Autodesk Fusion 360 part; units mm, degrees
(part 6 of 13)
  line L4448 (118.391, -108.231) -> (118.395, -108.209)
  line L4449 (123.628, -105.486) -> (123.648, -105.363)
  line L4450 (118.413, -108.169) -> (118.428, -108.142)
  line L4451 (133.306, -110.097) -> (133.194, -110.04)
  line L4452 (134.009, -109.5) -> (133.915, -109.438)
  line L4453 (133.194, -110.04) -> (133.106, -109.952)
  line L4454 (124.028, -105.086) -> (124.152, -105.106)
  line L4455 (133.665, -110.04) -> (133.553, -110.097)
  line L4456 (133.753, -109.952) -> (133.665, -110.04)
  line L4457 (119.458, -107.165) -> (123.205, -107.165)
  line L4458 (133.049, -109.84) -> (133.029, -109.717)
  line L4459 (133.194, -109.393) -> (133.306, -109.336)
  line L4460 (123.648, -105.363) -> (123.705, -105.251)
  line L4461 (134.224, -109.549) -> (134.224, -109.544)
  line L4462 (133.765, -109.235) -> (133.742, -109.183)
  line L4463 (134.144, -109.542) -> (134.009, -109.5)
  line L4464 (133.915, -109.438) -> (133.79, -109.553)
  line L4465 (133.106, -109.952) -> (133.049, -109.84)
  line L4466 (134.724, -109.549) -> (134.224, -109.549)
  line L4467 (133.029, -109.717) -> (133.049, -109.593)
  line L4468 (123.793, -105.163) -> (123.905, -105.106)
  line L4469 (133.049, -109.593) -> (133.106, -109.481)
  line L4470 (133.62, -109.37) -> (133.765, -109.235)
  line L4471 (133.553, -110.097) -> (133.429, -110.117)
  line L4472 (133.429, -110.117) -> (133.306, -110.097)
  line L4473 (133.829, -109.717) -> (133.81, -109.84)
  line L4474 (118.571, -110.489) -> (118.459, -110.433)
  line L4475 (133.81, -109.84) -> (133.753, -109.952)
  line L4476 (134.224, -109.544) -> (134.144, -109.542)
  line L4477 (133.106, -109.481) -> (133.194, -109.393)
  line L4478 (118.371, -110.344) -> (118.314, -110.233)
  line L4479 (133.553, -109.336) -> (133.62, -109.37)
  line L4480 (134.156, -108.053) -> (134.224, -108.054)
  line L4481 (133.806, -108.274) -> (133.9, -108.168)
  line L4482 (136.967, -108.279) -> (136.994, -108.293)
  line L4483 (123.705, -105.251) -> (123.793, -105.163)
  line L4484 (133.81, -109.593) -> (133.829, -109.717)
  line L4485 (123.905, -105.106) -> (124.028, -105.086)
  line L4486 (137.092, -108.839) -> (137.147, -108.839)
  line L4487 (134.02, -108.092) -> (134.156, -108.053)
  line L4488 (137.36, -108.659) -> (137.374, -108.677)
  line L4489 (133.724, -109.049) -> (133.724, -108.549)
  line L4490 (137.47, -108.851) -> (137.472, -108.859)
  line L4491 (137.147, -108.8) -> (136.854, -108.507)
  line L4492 (135.941, -108.257) -> (136.906, -108.257)
  line L4493 (133.724, -108.549) -> (133.725, -108.549)
  line L4494 (136.933, -108.26) -> (136.935, -108.261)
  line L4495 (135.598, -108.054) -> (135.734, -108.095)
  line L4496 (137.074, -108.851) -> (137.078, -108.845)
  line L4497 (133.725, -108.549) -> (133.724, -108.543)
  line L4498 (135.929, -108.26) -> (135.941, -108.257)
  line L4499 (136.928, -108.26) -> (136.933, -108.26)
  line L4500 (133.724, -108.543) -> (133.746, -108.403)
  line L4501 (136.018, -108.507) -> (136.024, -108.549)
  line L4502 (137.378, -108.683) -> (137.382, -108.688)
  line L4503 (133.742, -109.183) -> (133.725, -109.049)
  line L4504 (136.935, -108.261) -> (136.942, -108.262)
  line L4505 (133.725, -109.049) -> (133.724, -109.049)
  line L4506 (137.374, -108.677) -> (137.377, -108.68)
  line L4507 (137.377, -108.68) -> (137.378, -108.683)
  line L4508 (133.9, -108.168) -> (134.02, -108.092)
  line L4509 (133.746, -108.403) -> (133.806, -108.274)
  line L4510 (135.524, -108.054) -> (135.598, -108.054)
  line L4511 (134.224, -108.049) -> (134.724, -108.049)
  line L4512 (136, -109.201) -> (135.939, -109.328)
  line L4513 (137.072, -110.009) -> (137.072, -108.859)
  line L4514 (137.46, -110.027) -> (137.452, -110.029)
  line L4515 (134.224, -108.054) -> (134.224, -108.049)
  line L4516 (137.084, -108.84) -> (137.092, -108.839)
  line L4517 (135.853, -108.172) -> (135.929, -108.26)
  line L4518 (136.942, -108.262) -> (136.967, -108.279)
  line L4519 (137.074, -110.016) -> (137.072, -110.009)
  line L4520 (136.854, -108.507) -> (136.018, -108.507)
  line L4521 (134.724, -108.049) -> (134.724, -109.549)
  line L4522 (136.994, -108.293) -> (137.36, -108.659)
  line L4523 (137.092, -110.029) -> (137.084, -110.027)
  line L4524 (136.906, -108.257) -> (136.928, -108.26)
  line L4525 (137.078, -108.845) -> (137.084, -108.84)
  line L4526 (137.397, -108.839) -> (137.452, -108.839)
  line L4527 (137.078, -110.023) -> (137.074, -110.016)
  line L4528 (137.452, -110.029) -> (137.092, -110.029)
  line L4529 (129.83, -106.256) -> (129.693, -106.294)
  line L4530 (135.723, -109.508) -> (135.586, -109.545)
  line L4531 (129.631, -104.798) -> (129.631, -104.803)
  line L4532 (137.472, -108.859) -> (137.472, -110.009)
  line L4533 (137.072, -108.859) -> (137.074, -108.851)
  line L4534 (137.147, -108.839) -> (137.147, -108.8)
  line L4535 (137.084, -110.027) -> (137.078, -110.023)
  line L4536 (137.388, -108.718) -> (137.397, -108.748)
  line L4537 (130.888, -105.969) -> (130.87, -105.977)
  line L4538 (135.024, -108.049) -> (135.524, -108.049)
  line L4539 (135.524, -109.544) -> (135.524, -109.549)
  line L4540 (129.951, -106.182) -> (129.83, -106.256)
  line L4541 (137.382, -108.688) -> (137.388, -108.718)
  line L4542 (137.466, -108.845) -> (137.47, -108.851)
  line L4543 (137.466, -110.023) -> (137.46, -110.027)
  line L4544 (135.524, -108.049) -> (135.524, -108.054)
  line L4545 (130.927, -105.936) -> (130.888, -105.969)
  line L4546 (135.024, -109.549) -> (135.024, -108.049)
  line L4547 (136.024, -108.549) -> (136.024, -109.049)
  line L4548 (129.131, -106.298) -> (129.131, -104.798)
  line L4549 (137.47, -110.016) -> (137.466, -110.023)
  line L4550 (130.968, -105.905) -> (130.927, -105.936)
  line L4551 (130.669, -106.04) -> (130.619, -106.048)
  line L4552 (130.759, -106.028) -> (130.739, -106.03)
  line L4553 (135.843, -109.433) -> (135.723, -109.508)
  line L4554 (130.805, -106.006) -> (130.759, -106.028)
  line L4555 (136.024, -109.049) -> (136.024, -109.061)
  line L4556 (129.693, -106.294) -> (129.631, -106.293)
  line L4557 (137.46, -108.84) -> (137.466, -108.845)
  line L4558 (129.631, -106.293) -> (129.631, -106.298)
  line L4559 (130.853, -105.989) -> (130.805, -106.006)
  line L4560 (130.739, -106.03) -> (130.72, -106.037)
  line L4561 (136.024, -109.061) -> (136, -109.201)
  line L4562 (137.452, -108.839) -> (137.46, -108.84)
  line L4563 (135.524, -109.549) -> (135.024, -109.549)
  line L4564 (130.972, -105.901) -> (130.968, -105.905)
  line L4565 (137.397, -108.748) -> (137.397, -108.839)
  line L4566 (137.472, -110.009) -> (137.47, -110.016)
  line L4567 (135.939, -109.328) -> (135.843, -109.433)
  line L4568 (135.586, -109.545) -> (135.524, -109.544)
  line L4569 (129.131, -104.798) -> (129.631, -104.798)
  line L4570 (130.046, -106.077) -> (129.951, -106.182)
  line L4571 (130.87, -105.977) -> (130.853, -105.989)
  line L4572 (130.411, -105.048) -> (131.072, -104.387)
  line L4573 (138.032, -108.702) -> (138.038, -108.732)
  line L4574 (142.55, -97.9698) -> (142.58, -98.011)
  line L4575 (130.061, -105.048) -> (130.411, -105.048)
  line L4576 (138.11, -108.84) -> (138.116, -108.845)
  line L4577 (131.072, -106.624) -> (131.072, -105.801)
  line L4578 (137.724, -108.851) -> (137.728, -108.845)
  line L4579 (138.038, -108.732) -> (138.047, -108.761)
  line L4580 (131.582, -106.402) -> (132.014, -106.834)
  line L4581 (129.96, -104.921) -> (130.052, -105.028)
  line L4582 (131.582, -106.044) -> (131.582, -106.402)
  line L4583 (135.012, -106.044) -> (131.582, -106.044)
  line L4584 (136.208, -106.871) -> (138.01, -108.673)
  line L4585 (138.116, -108.845) -> (138.12, -108.851)
  line L4586 (136.149, -106.839) -> (136.155, -106.84)
  line L4587 (138.047, -108.839) -> (138.102, -108.839)
  line L4588 (136.181, -106.856) -> (136.208, -106.871)
  line L4589 (138.024, -108.691) -> (138.027, -108.694)
  line L4590 (131.072, -104.387) -> (131.072, -100.204)
  line L4591 (136.155, -106.84) -> (136.181, -106.856)
  line L4592 (130.619, -106.048) -> (130.06, -106.048)
  line L4593 (138.01, -108.673) -> (138.024, -108.691)
  line L4594 (138.102, -108.839) -> (138.11, -108.84)
  line L4595 (138.12, -108.851) -> (138.122, -108.859)
  line L4596 (130.06, -106.048) -> (130.046, -106.077)
  line L4597 (130.72, -106.037) -> (130.669, -106.04)
  line L4598 (130.052, -105.028) -> (130.061, -105.048)
  line L4599 (136.142, -106.838) -> (136.147, -106.837)
  line L4600 (131.072, -105.801) -> (130.972, -105.901)
  line L4601 (129.705, -104.803) -> (129.841, -104.844)
  line L4602 (131.072, -100.204) -> (135.012, -100.204)
  line L4603 (129.631, -106.298) -> (129.131, -106.298)
  line L4604 (136.147, -106.837) -> (136.149, -106.839)
  line L4605 (138.027, -108.694) -> (138.028, -108.697)
  line L4606 (129.631, -104.803) -> (129.705, -104.803)
  line L4607 (138.028, -108.697) -> (138.032, -108.702)
  line L4608 (136.12, -106.834) -> (136.142, -106.838)
  line L4609 (132.014, -106.834) -> (136.12, -106.834)
  line L4610 (138.047, -108.761) -> (138.047, -108.839)
  line L4611 (135.012, -100.204) -> (135.012, -106.044)
  line L4612 (129.841, -104.844) -> (129.96, -104.921)
  line L4613 (138.122, -110.009) -> (138.12, -110.016)
  line L4614 (143.297, -107.059) -> (140.488, -107.059)
  line L4615 (142.546, -97.9655) -> (142.55, -97.9698)
  line L4616 (138.77, -108.851) -> (138.772, -108.859)
  line L4617 (142.651, -98.1322) -> (142.672, -98.1787)
  line L4618 (142.692, -98.319) -> (142.692, -100.204)
  line L4619 (131.963, -107.084) -> (131.941, -107.081)
  line L4620 (138.102, -110.029) -> (137.742, -110.029)
  line L4621 (137.724, -110.016) -> (137.722, -110.009)
  line L4622 (137.722, -110.009) -> (137.722, -108.859)
  line L4623 (137.734, -110.027) -> (137.728, -110.023)
  line L4624 (137.797, -108.839) -> (137.797, -108.813)
  line L4625 (131.936, -107.082) -> (131.933, -107.08)
  line L4626 (136.068, -107.084) -> (131.963, -107.084)
  line L4627 (137.728, -110.023) -> (137.724, -110.016)
  line L4628 (138.122, -108.859) -> (138.122, -110.009)
  line L4629 (131.941, -107.081) -> (131.936, -107.082)
  line L4630 (137.742, -108.839) -> (137.797, -108.839)
  line L4631 (138.11, -110.027) -> (138.102, -110.029)
  line L4632 (137.797, -108.813) -> (136.068, -107.084)
  line L4633 (137.722, -108.859) -> (137.724, -108.851)
  line L4634 (131.45, -106.624) -> (131.072, -106.624)
  line L4635 (142.672, -98.1787) -> (142.675, -98.1986)
  line L4636 (144.162, -106.624) -> (143.784, -106.624)
  line L4637 (142.622, -98.068) -> (142.634, -98.0843)
  line L4638 (131.933, -107.08) -> (131.927, -107.079)
  line L4639 (137.734, -108.84) -> (137.742, -108.839)
  line L4640 (143.362, -107.04) -> (143.357, -107.044)
  line L4641 (142.58, -98.011) -> (142.613, -98.0496)
  line L4642 (131.927, -107.079) -> (131.901, -107.063)
  line L4643 (138.12, -110.016) -> (138.116, -110.023)
  line L4644 (142.682, -98.2176) -> (142.685, -98.2685)
  line L4645 (131.901, -107.063) -> (131.874, -107.048)
  line L4646 (142.634, -98.0843) -> (142.651, -98.1322)
  line L4647 (144.162, -100.204) -> (144.162, -106.624)
  line L4648 (138.116, -110.023) -> (138.11, -110.027)
  line L4649 (142.613, -98.0496) -> (142.622, -98.068)
  line L4650 (143.784, -106.624) -> (143.386, -107.022)
  line L4651 (143.365, -107.039) -> (143.362, -107.04)
  line L4652 (131.874, -107.048) -> (131.45, -106.624)
  line L4653 (137.742, -110.029) -> (137.734, -110.027)
  line L4654 (138.766, -108.845) -> (138.77, -108.851)
  line L4655 (137.728, -108.845) -> (137.734, -108.84)
  line L4656 (143.357, -107.044) -> (143.327, -107.05)
  line L4657 (94.627, -94.7818) -> (92.227, -94.7818)
  line L4658 (89.8672, -95.377) -> (89.8704, -95.355)
  line L4659 (89.8704, -95.355) -> (89.8701, -95.3504)
  line L4660 (91.5604, -94.2021) -> (91.6036, -94.2868)
  line L4661 (89.9038, -97.472) -> (89.8905, -97.4542)
  line L4662 (90.8436, -94.3488) -> (90.8518, -94.3427)
  line L4663 (91.4719, -94.1136) -> (91.5604, -94.2021)
  line L4664 (137.966, -94.6836) -> (137.963, -94.6327)
  line L4665 (140.488, -107.059) -> (138.709, -108.839)
  line L4666 (91.6036, -94.2868) -> (92.227, -94.2868)
  line L4667 (89.8714, -95.3479) -> (89.8723, -95.3415)
  line L4668 (143.327, -107.05) -> (143.297, -107.059)
  line L4669 (89.8701, -95.3504) -> (89.8714, -95.3479)
  line L4670 (90.9132, -94.2021) -> (91.0017, -94.1136)
  line L4671 (142.685, -98.2685) -> (142.692, -98.319)
  line L4672 (142.692, -100.204) -> (144.162, -100.204)
  line L4673 (92.227, -94.2868) -> (92.227, -94.0418)
  line L4674 (143.368, -107.036) -> (143.365, -107.039)
  line L4675 (91.0017, -94.1136) -> (91.1132, -94.0568)
  line L4676 (89.8862, -97.4484) -> (89.8823, -97.4432)
  line L4677 (92.227, -94.5368) -> (91.621, -94.5368)
  line L4678 (89.8823, -97.4432) -> (89.8759, -97.4131)
  line L4679 (89.8672, -97.3836) -> (89.8672, -95.377)
  line L4680 (143.386, -107.022) -> (143.368, -107.036)
  line L4681 (138.76, -108.84) -> (138.766, -108.845)
  line L4682 (89.8905, -97.4542) -> (89.887, -97.4511)
  line L4683 (91.2368, -94.0372) -> (91.3604, -94.0568)
  line L4684 (90.8518, -94.3427) -> (90.8564, -94.3136)
  line L4685 (89.8759, -97.4131) -> (89.8672, -97.3836)
  line L4686 (92.227, -94.7818) -> (92.227, -94.5368)
  line L4687 (91.9866, -99.5548) -> (89.9038, -97.472)
  line L4688 (90.8564, -94.3136) -> (90.9132, -94.2021)
  line L4689 (92.227, -94.0418) -> (94.627, -94.0418)
  line L4690 (89.8723, -95.3415) -> (89.889, -95.3156)
  line L4691 (138.709, -108.839) -> (138.752, -108.839)
  line L4692 (91.1132, -94.0568) -> (91.2368, -94.0372)
  line L4693 (138.752, -108.839) -> (138.76, -108.84)
  line L4694 (91.3604, -94.0568) -> (91.4719, -94.1136)
  line L4695 (89.887, -97.4511) -> (89.8862, -97.4484)
  line L4696 (142.675, -98.1986) -> (142.682, -98.2176)
  line L4697 (94.627, -94.0418) -> (94.627, -94.7818)
  line L4698 (89.889, -95.3156) -> (89.9038, -95.2886)
  line L4699 (89.9038, -95.2886) -> (90.8436, -94.3488)
  line L4700 (117.818, -108.828) -> (117.873, -108.828)
  line L4701 (117.893, -108.848) -> (117.893, -109.998)
  line L4702 (137.963, -94.6327) -> (137.955, -94.5822)
  line L4703 (117.873, -110.018) -> (117.513, -110.018)
  line L4704 (138.102, -94.9358) -> (138.098, -94.9314)
  line L4705 (137.646, -94.1647) -> (137.607, -94.198)
  line L4706 (141.692, -98.5261) -> (138.102, -94.9358)
  line L4707 (143.652, -106.402) -> (143.652, -106.044)
  line L4708 (143.652, -106.044) -> (140.222, -106.044)
  line L4709 (137.573, -94.2183) -> (137.525, -94.2356)
  line L4710 (137.975, -94.7225) -> (137.973, -94.7026)
  line L4711 (141.692, -100.204) -> (141.692, -98.5261)
  line L4712 (137.955, -94.5822) -> (137.955, -93.8663)
  line L4713 (130.052, -94.2768) -> (123.283, -101.045)
  line L4714 (137.997, -94.769) -> (137.975, -94.7225)
  line L4715 (138.014, -94.8169) -> (137.997, -94.769)
  line L4716 (137.691, -94.1304) -> (137.687, -94.1346)
  line L4717 (138.026, -94.8332) -> (138.014, -94.8169)
  line L4718 (138.098, -94.9314) -> (138.067, -94.8902)
  line L4719 (138.034, -94.8516) -> (138.026, -94.8332)
  line L4720 (137.478, -94.2567) -> (137.458, -94.2596)
  line L4721 (137.607, -94.198) -> (137.589, -94.2064)
  line L4722 (117.881, -110.017) -> (117.873, -110.018)
  line L4723 (117.499, -108.834) -> (117.506, -108.83)
  line L4724 (117.893, -109.998) -> (117.892, -110.006)
  line L4725 (137.338, -94.2768) -> (130.052, -94.2768)
  line L4726 (117.495, -108.841) -> (117.499, -108.834)
  line L4727 (137.973, -94.7026) -> (137.966, -94.6836)
  line L4728 (140.222, -100.204) -> (141.692, -100.204)
  line L4729 (137.458, -94.2596) -> (137.439, -94.2664)
  line L4730 (137.955, -93.8663) -> (137.691, -94.1304)
  line L4731 (137.388, -94.2696) -> (137.338, -94.2768)
  line L4732 (138.067, -94.8902) -> (138.034, -94.8516)
  line L4733 (137.589, -94.2064) -> (137.573, -94.2183)
  line L4734 (137.525, -94.2356) -> (137.478, -94.2567)
  line L4735 (137.439, -94.2664) -> (137.388, -94.2696)
  line L4736 (122.699, -106.912) -> (122.696, -106.913)
  line L4737 (117.887, -108.834) -> (117.892, -108.841)
  line L4738 (122.691, -106.917) -> (122.661, -106.923)
  line L4739 (117.493, -108.848) -> (117.495, -108.841)
  line L4740 (140.222, -106.044) -> (140.222, -100.204)
  line L4741 (123.283, -101.045) -> (123.283, -106.613)
  line L4742 (137.687, -94.1346) -> (137.646, -94.1647)
  line L4743 (117.506, -110.017) -> (117.499, -110.012)
  line L4744 (122.661, -106.923) -> (122.631, -106.932)
  line L4745 (117.568, -108.418) -> (117.571, -108.396)
  line L4746 (122.721, -100.193) -> (129.491, -93.4232)
  line L4747 (119.274, -106.691) -> (119.304, -106.682)
  line L4748 (122.696, -106.913) -> (122.691, -106.917)
  line L4749 (117.892, -110.006) -> (117.887, -110.012)
  line L4750 (119.236, -106.702) -> (119.239, -106.701)
  line L4751 (129.496, -93.419) -> (129.537, -93.3889)
  line L4752 (123.002, -106.613) -> (122.72, -106.895)
  line L4753 (123.283, -106.613) -> (123.002, -106.613)
  line L4754 (129.491, -93.4232) -> (129.496, -93.419)
  line L4755 (117.513, -110.018) -> (117.506, -110.017)
  line L4756 (117.571, -108.396) -> (117.571, -108.391)
  line L4757 (117.818, -108.469) -> (117.818, -108.828)
  line L4758 (117.571, -108.391) -> (117.572, -108.388)
  line L4759 (122.631, -106.932) -> (119.356, -106.932)
  line L4760 (119.343, -100.193) -> (122.721, -100.193)
  line L4761 (117.892, -108.841) -> (117.893, -108.848)
  line L4762 (117.568, -108.828) -> (117.568, -108.418)
  line L4763 (117.506, -108.83) -> (117.513, -108.828)
  line L4764 (117.513, -108.828) -> (117.568, -108.828)
  line L4765 (129.575, -93.3556) -> (129.594, -93.3472)
  line L4766 (117.887, -110.012) -> (117.881, -110.017)
  line L4767 (122.702, -106.909) -> (122.699, -106.912)
  line L4768 (129.594, -93.3472) -> (129.61, -93.3353)
  line L4769 (117.493, -109.998) -> (117.493, -108.848)
  line L4770 (117.573, -108.382) -> (117.59, -108.356)
  line L4771 (129.61, -93.3353) -> (129.658, -93.318)
  line L4772 (117.495, -110.006) -> (117.493, -109.998)
  line L4773 (122.72, -106.895) -> (122.702, -106.909)
  line L4774 (129.537, -93.3889) -> (129.575, -93.3556)
  line L4775 (122.773, -106.033) -> (119.343, -106.033)
  line L4776 (129.658, -93.318) -> (129.704, -93.2969)
  line L4777 (117.873, -108.828) -> (117.881, -108.83)
  line L4778 (119.343, -106.033) -> (119.343, -100.193)
  line L4779 (117.499, -110.012) -> (117.495, -110.006)
  line L4780 (117.881, -108.83) -> (117.887, -108.834)
  line L4781 (117.572, -108.388) -> (117.573, -108.382)
  line L4782 (122.579, -106.682) -> (122.773, -106.488)
  line L4783 (129.704, -93.2969) -> (129.724, -93.294)
  line L4784 (119.356, -106.932) -> (117.818, -108.469)
  line L4785 (137.955, -85.8813) -> (137.162, -85.088)
  line L4786 (117.605, -108.329) -> (119.215, -106.719)
  line L4787 (122.773, -106.488) -> (122.773, -106.033)
  line L4788 (135.862, -82.6562) -> (136.017, -82.6358)
  line L4789 (129.743, -93.2872) -> (129.794, -93.284)
  line L4790 (140.196, -81.9356) -> (140.136, -81.7909)
  line L4791 (135.862, -83.8154) -> (135.717, -83.7554)
  line L4792 (140.538, -71.1574) -> (140.704, -71.1772)
  line L4793 (136.601, -83.1125) -> (137.832, -84.3433)
  line L4794 (137.162, -85.088) -> (137.162, -85.088)
  line L4795 (129.794, -93.284) -> (129.845, -93.2768)
  line L4796 (136.441, -82.8115) -> (136.537, -82.9358)
  line L4797 (135.437, -83.3911) -> (135.417, -83.2358)
  line L4798 (135.717, -82.7162) -> (135.862, -82.6562)
  line L4799 (135.437, -83.0805) -> (135.497, -82.9358)
  line L4800 (135.417, -83.2358) -> (135.437, -83.0805)
  line L4801 (129.724, -93.294) -> (129.743, -93.2872)
  line L4802 (119.244, -106.697) -> (119.274, -106.691)
  line L4803 (119.304, -106.682) -> (122.579, -106.682)
  line L4804 (117.59, -108.356) -> (117.605, -108.329)
  line L4805 (119.239, -106.701) -> (119.244, -106.697)
  line L4806 (136.317, -82.7162) -> (136.441, -82.8115)
  line L4807 (129.845, -93.2768) -> (137.131, -93.2768)
  line L4808 (137.162, -85.088) -> (135.894, -83.8196)
  line L4809 (119.233, -106.705) -> (119.236, -106.702)
  line L4810 (140.116, -81.6356) -> (140.136, -81.4803)
  line L4811 (136.597, -83.0805) -> (136.601, -83.1125)
  line L4812 (137.131, -93.2768) -> (137.955, -92.4521)
  line L4813 (135.497, -82.9358) -> (135.593, -82.8115)
  line L4814 (137.955, -92.4521) -> (137.955, -85.8813)
  line L4815 (119.215, -106.719) -> (119.233, -106.705)
  line L4816 (135.894, -83.8196) -> (135.862, -83.8154)
  line L4817 (140.136, -81.7909) -> (140.116, -81.6356)
  line L4818 (135.593, -82.8115) -> (135.717, -82.7162)
  line L4819 (136.537, -82.9358) -> (136.597, -83.0805)
  line L4820 (140.136, -81.4803) -> (140.196, -81.3356)
  line L4821 (135.717, -83.7554) -> (135.593, -83.6601)
  line L4822 (135.497, -83.5358) -> (135.437, -83.3911)
  line L4823 (135.593, -83.6601) -> (135.497, -83.5358)
  line L4824 (137.832, -84.3433) -> (140.215, -81.9598)
  line L4825 (140.215, -81.9598) -> (140.196, -81.9356)
  line L4826 (136.017, -82.6358) -> (136.172, -82.6562)
  line L4827 (136.172, -82.6562) -> (136.317, -82.7162)
  line L4828 (140.658, -81.0432) -> (140.716, -81.0356)
  line L4829 (140.658, -72.6444) -> (140.658, -81.0432)
  line L4830 (140.392, -82.1366) -> (138.008, -84.52)
  line L4831 (140.871, -81.056) -> (141.016, -81.116)
  line L4832 (140.071, -71.3164) -> (140.214, -71.2288)
  line L4833 (141.316, -81.6356) -> (141.296, -81.7909)
  line L4834 (141.016, -82.1552) -> (140.871, -82.2152)
  line L4835 (139.8, -72.0633) -> (139.783, -71.8969)
  line L4836 (140.195, -72.5768) -> (140.055, -72.4853)
  line L4837 (140.055, -72.4853) -> (139.939, -72.365)
  line L4838 (141.108, -72.3895) -> (140.987, -72.5048)
  line L4839 (140.862, -71.2333) -> (141.003, -71.3229)
  line L4840 (140.214, -71.2288) -> (140.372, -71.1749)
  line L4841 (139.939, -72.365) -> (139.852, -72.222)
  line L4842 (140.372, -71.1749) -> (140.538, -71.1574)
  line L4843 (140.716, -82.2356) -> (140.561, -82.2152)
  line L4844 (141.283, -71.9283) -> (141.26, -72.0939)
  line L4845 (141.121, -71.4415) -> (141.209, -71.5833)
  line L4846 (140.704, -71.1772) -> (140.862, -71.2333)
  line L4847 (141.264, -71.7412) -> (141.283, -71.9074)
  line L4848 (140.843, -72.5904) -> (140.684, -72.6421)
  line L4849 (141.003, -71.3229) -> (141.121, -71.4415)
  line L4850 (141.283, -71.9074) -> (141.283, -71.9283)
  line L4851 (140.352, -72.6351) -> (140.195, -72.5768)
  line L4852 (138.885, -85.4232) -> (138.897, -85.4395)
  line L4853 (140.292, -81.2113) -> (140.408, -81.122)
  line L4854 (139.804, -71.731) -> (139.861, -71.5739)
  line L4855 (141.296, -81.7909) -> (141.236, -81.9356)
  line L4856 (141.236, -81.9356) -> (141.14, -82.0599)
  line L4857 (139.861, -71.5739) -> (139.952, -71.4334)
  line L4858 (139.852, -72.222) -> (139.8, -72.0633)
  line L4859 (138.809, -85.3206) -> (138.813, -85.325)
  line L4860 (141.14, -82.0599) -> (141.016, -82.1552)
  line L4861 (140.987, -72.5048) -> (140.843, -72.5904)
  line L4862 (141.2, -72.2502) -> (141.108, -72.3895)
  line L4863 (141.209, -71.5833) -> (141.264, -71.7412)
  line L4864 (140.408, -72.6427) -> (140.352, -72.6351)
  line L4865 (140.408, -81.122) -> (140.408, -72.6427)
  line L4866 (140.684, -72.6421) -> (140.658, -72.6444)
  line L4867 (141.26, -72.0939) -> (141.2, -72.2502)
  line L4868 (139.783, -71.8969) -> (139.804, -71.731)
  line L4869 (140.196, -81.3356) -> (140.292, -81.2113)
  line L4870 (139.952, -71.4334) -> (140.071, -71.3164)
  line L4871 (138.955, -94.3751) -> (142.546, -97.9655)
  line L4872 (140.716, -81.0356) -> (140.871, -81.056)
  line L4873 (138.955, -85.6742) -> (138.955, -94.3751)
  line L4874 (106.759, -99.937) -> (106.459, -99.937)
  line L4875 (106.059, -100.537) -> (106.059, -99.937)
  line L4876 (138.813, -85.325) -> (138.843, -85.3662)
  line L4877 (107.059, -98.587) -> (107.059, -98.437)
  line L4878 (141.016, -81.116) -> (141.14, -81.2113)
  line L4879 (108.059, -99.937) -> (107.059, -99.937)
  line L4880 (107.059, -99.787) -> (106.759, -99.787)
  line L4881 (106.059, -99.937) -> (105.759, -99.937)
  line L4882 (138.935, -85.5339) -> (138.938, -85.5538)
  line L4883 (141.14, -81.2113) -> (141.236, -81.3356)
  line L4884 (140.561, -82.2152) -> (140.416, -82.1552)
  line L4885 (107.059, -99.937) -> (107.059, -99.787)
  line L4886 (106.494, -101.202) -> (106.382, -101.259)
  line L4887 (106.023, -100.555) -> (106.059, -100.537)
  line L4888 (105.878, -101.002) -> (105.859, -100.878)
  line L4889 (105.878, -100.755) -> (105.935, -100.643)
  line L4890 (138.008, -84.52) -> (138.809, -85.3206)
  line L4891 (138.945, -85.5728) -> (138.948, -85.6237)
  line L4892 (138.914, -85.4874) -> (138.935, -85.5339)
  line L4893 (105.759, -99.937) -> (105.759, -98.437)
  line L4894 (106.135, -101.259) -> (106.023, -101.202)
  line L4895 (138.938, -85.5538) -> (138.945, -85.5728)
  line L4896 (106.459, -99.937) -> (106.459, -100.537)
  line L4897 (106.759, -98.587) -> (107.059, -98.587)
  line L4898 (138.843, -85.3662) -> (138.877, -85.4048)
  line L4899 (141.236, -81.3356) -> (141.296, -81.4803)
  line L4900 (106.759, -98.437) -> (106.759, -98.587)
  line L4901 (106.639, -100.755) -> (106.659, -100.878)
  line L4902 (141.296, -81.4803) -> (141.316, -81.6356)
  line L4903 (138.877, -85.4048) -> (138.885, -85.4232)
  line L4904 (138.897, -85.4395) -> (138.914, -85.4874)
  line L4905 (140.871, -82.2152) -> (140.716, -82.2356)
  line L4906 (105.859, -100.878) -> (105.878, -100.755)
  line L4907 (105.759, -98.437) -> (106.759, -98.437)
  line L4908 (106.659, -100.878) -> (106.639, -101.002)
  line L4909 (106.459, -100.537) -> (106.494, -100.555)
  line L4910 (140.416, -82.1552) -> (140.392, -82.1366)
  line L4911 (105.935, -100.643) -> (106.023, -100.555)
  line L4912 (138.948, -85.6237) -> (138.955, -85.6742)
  line L4913 (116.849, -108.834) -> (116.856, -108.83)
  line L4914 (106.759, -99.787) -> (106.759, -99.937)
  line L4915 (114.133, -106.033) -> (110.703, -106.033)
  line L4916 (108.254, -98.7057) -> (108.274, -98.7088)
  line L4917 (108.384, -98.7605) -> (108.402, -98.7691)
  line L4918 (105.935, -101.114) -> (105.878, -101.002)
  line L4919 (108.32, -98.7305) -> (108.368, -98.7484)
  line L4920 (115.571, -106.761) -> (115.574, -106.762)
  line L4921 (108.274, -98.7088) -> (108.32, -98.7305)
  line L4922 (108.134, -98.687) -> (108.184, -98.6949)
  line L4923 (108.235, -98.6987) -> (108.254, -98.7057)
  line L4924 (115.633, -106.795) -> (117.132, -108.293)
  line L4925 (115.58, -106.763) -> (115.606, -106.78)
  line L4926 (106.582, -101.114) -> (106.494, -101.202)
  line L4927 (117.132, -108.293) -> (117.145, -108.311)
  line L4928 (106.259, -101.278) -> (106.135, -101.259)
  line L4929 (106.494, -100.555) -> (106.582, -100.643)
  line L4930 (106.582, -100.643) -> (106.639, -100.755)
  line L4931 (106.639, -101.002) -> (106.582, -101.114)
  line L4932 (106.382, -101.259) -> (106.259, -101.278)
  line L4933 (108.059, -98.687) -> (108.128, -98.687)
  line L4934 (107.059, -98.437) -> (108.059, -98.437)
  line L4935 (108.402, -98.7691) -> (108.441, -98.8029)
  line L4936 (110.703, -106.033) -> (110.703, -106.392)
  line L4937 (108.128, -98.687) -> (108.134, -98.687)
  line L4938 (108.059, -99.8249) -> (108.059, -99.937)
  line L4939 (110.193, -100.545) -> (110.193, -100.193)
  line L4940 (106.023, -101.202) -> (105.935, -101.114)
  line L4941 (111.07, -106.758) -> (115.545, -106.758)
  line L4942 (108.481, -98.8334) -> (110.193, -100.545)
  line L4943 (115.545, -106.758) -> (115.567, -106.761)
  line L4944 (110.193, -100.193) -> (114.133, -100.193)
  line L4945 (115.567, -106.761) -> (115.571, -106.761)
  line L4946 (114.133, -100.193) -> (114.133, -106.033)
  line L4947 (115.606, -106.78) -> (115.633, -106.795)
  line L4948 (115.574, -106.762) -> (115.58, -106.763)
  line L4949 (108.184, -98.6949) -> (108.235, -98.6987)
  line L4950 (108.441, -98.8029) -> (108.481, -98.8334)
  line L4951 (108.059, -98.437) -> (108.059, -98.687)
  line L4952 (117.145, -108.311) -> (117.148, -108.314)
  line L4953 (117.148, -108.314) -> (117.149, -108.317)
  line L4954 (108.368, -98.7484) -> (108.384, -98.7605)
  line L4955 (110.703, -106.392) -> (111.07, -106.758)
  line L4956 (110.989, -107.004) -> (110.983, -107.003)
  line L4957 (117.242, -108.841) -> (117.243, -108.848)
  line L4958 (145.193, -107.55) -> (145.281, -107.639)
  line L4959 (116.918, -108.434) -> (115.493, -107.008)
  line L4960 (147.004, -109.451) -> (146.923, -109.505)
  line L4961 (116.845, -108.841) -> (116.849, -108.834)
  line L4962 (146.923, -108.418) -> (147.004, -108.473)
  line L4963 (145.401, -109.451) -> (145.346, -109.37)
  line L4964 (117.243, -108.848) -> (117.243, -109.998)
  line L4965 (117.168, -108.828) -> (117.223, -108.828)
  line L4966 (117.237, -108.834) -> (117.242, -108.841)
  line L4967 (110.193, -101.96) -> (108.059, -99.8249)
  line L4968 (117.242, -110.006) -> (117.237, -110.012)
  line L4969 (117.153, -108.322) -> (117.16, -108.352)
  line L4970 (111.018, -107.008) -> (110.996, -107.005)
  line L4971 (116.845, -110.006) -> (116.843, -109.998)
  line L4972 (116.843, -109.998) -> (116.843, -108.848)
  line L4973 (117.231, -110.017) -> (117.223, -110.018)
  line L4974 (117.231, -108.83) -> (117.237, -108.834)
  line L4975 (110.572, -106.613) -> (110.193, -106.613)
  line L4976 (116.849, -110.012) -> (116.845, -110.006)
  line L4977 (115.493, -107.008) -> (111.018, -107.008)
  line L4978 (116.843, -108.848) -> (116.845, -108.841)
  line L4979 (147.058, -109.37) -> (147.004, -109.451)
  line L4980 (117.16, -108.352) -> (117.168, -108.382)
  line L4981 (110.996, -107.005) -> (110.992, -107.005)
  line L4982 (116.863, -108.828) -> (116.918, -108.828)
  line L4983 (116.856, -108.83) -> (116.863, -108.828)
  line L4984 (116.863, -110.018) -> (116.856, -110.017)
  line L4985 (110.193, -106.613) -> (110.193, -101.96)
  line L4986 (145.376, -107.785) -> (145.99, -108.399)
  line L4987 (117.149, -108.317) -> (117.153, -108.322)
  line L4988 (147.077, -109.274) -> (147.058, -109.37)
  line L4989 (145.99, -108.399) -> (146.827, -108.399)
  line L4990 (117.237, -110.012) -> (117.231, -110.017)
  line L4991 (145.341, -107.765) -> (145.349, -107.771)
  line L4992 (117.223, -110.018) -> (116.863, -110.018)
  line L4993 (117.168, -108.382) -> (117.168, -108.828)
  line L4994 (110.992, -107.005) -> (110.989, -107.004)
  line L4995 (117.223, -108.828) -> (117.231, -108.83)
  line L4996 (116.856, -110.017) -> (116.849, -110.012)
  line L4997 (116.918, -108.828) -> (116.918, -108.434)
  line L4998 (117.243, -109.998) -> (117.242, -110.006)
  line L4999 (142.886, -109.451) -> (142.832, -109.37)
  line L5000 (145.401, -108.473) -> (145.482, -108.418)
  line L5001 (144.544, -109.37) -> (144.49, -109.451)
  line L5002 (145.577, -108.399) -> (145.637, -108.399)
  line L5003 (145.577, -109.524) -> (145.482, -109.505)
  line L5004 (147.058, -108.554) -> (147.077, -108.649)
  line L5005 (110.983, -107.003) -> (110.957, -106.986)
  line L5006 (147.077, -108.649) -> (147.077, -109.274)
  line L5007 (145.281, -108.109) -> (145.193, -108.197)
  line L5008 (145.349, -107.771) -> (145.376, -107.785)
  line L5009 (145.327, -109.274) -> (145.327, -108.649)
  line L5010 (144.05, -108.399) -> (144.313, -108.399)
  line L5011 (106.759, -99.387) -> (107.059, -99.387)
  line L5012 (144.634, -108.109) -> (144.578, -107.999)
  line L5013 (107.059, -98.987) -> (106.759, -98.987)
  line L5014 (145.346, -109.37) -> (145.327, -109.274)
  line L5015 (145.081, -107.493) -> (145.193, -107.55)
  line L5016 (144.49, -108.473) -> (144.544, -108.554)
  line L5017 (144.723, -108.197) -> (144.634, -108.109)
  line L5018 (145.281, -107.639) -> (145.338, -107.75)
  line L5019 (144.408, -109.505) -> (144.313, -109.524)
  line L5020 (145.346, -108.554) -> (145.401, -108.473)
  line L5021 (106.759, -98.987) -> (106.759, -99.387)
  line L5022 (146.827, -109.524) -> (145.577, -109.524)
  line L5023 (144.49, -109.451) -> (144.408, -109.505)
  line L5024 (144.834, -108.254) -> (144.723, -108.197)
  line L5025 (144.544, -108.554) -> (144.563, -108.649)
  line L5026 (107.059, -99.387) -> (107.059, -98.987)
  line L5027 (144.563, -108.649) -> (144.563, -109.274)
  line L5028 (146.923, -109.505) -> (146.827, -109.524)
  line L5029 (142.967, -109.505) -> (142.886, -109.451)
  line L5030 (145.081, -108.254) -> (144.958, -108.274)
  line L5031 (144.958, -108.274) -> (144.834, -108.254)
  line L5032 (145.482, -109.505) -> (145.401, -109.451)
  line L5033 (146.827, -108.399) -> (146.923, -108.418)
  line L5034 (145.637, -108.399) -> (145.303, -108.066)
  line L5035 (147.004, -108.473) -> (147.058, -108.554)
  line L5036 (144.451, -107.999) -> (144.05, -108.399)
  line L5037 (145.338, -107.75) -> (145.341, -107.765)
  line L5038 (110.957, -106.986) -> (110.93, -106.972)
  line L5039 (110.93, -106.972) -> (110.572, -106.613)
  line L5040 (145.327, -108.649) -> (145.346, -108.554)
  line L5041 (143.063, -109.524) -> (142.967, -109.505)
  line L5042 (142.813, -109.274) -> (142.813, -108.649)
  line L5043 (144.578, -107.749) -> (144.634, -107.639)
  line L5044 (130.654, -107.595) -> (130.766, -107.652)
  line L5045 (144.311, -107.785) -> (144.328, -107.772)
  line L5046 (142.813, -108.649) -> (142.832, -108.554)
  line L5047 (142.832, -109.37) -> (142.813, -109.274)
  line L5048 (144.339, -107.764) -> (144.369, -107.757)
  line L5049 (131.567, -108.399) -> (132.578, -108.399)
  line L5050 (144.563, -109.274) -> (144.544, -109.37)
  line L5051 (131.028, -107.872) -> (131.055, -107.887)
  line L5052 (144.328, -107.772) -> (144.331, -107.769)
  line L5053 (144.958, -107.474) -> (145.081, -107.493)
  line L5054 (142.832, -108.554) -> (142.886, -108.473)
  line L5055 (143.697, -108.399) -> (144.311, -107.785)
  line L5056 (144.634, -107.639) -> (144.723, -107.55)
  line L5057 (130.989, -107.854) -> (130.993, -107.853)
  line L5058 (130.966, -107.85) -> (130.989, -107.854)
  line L5059 (129.979, -108.399) -> (130.114, -108.399)
  line L5060 (131.002, -107.856) -> (131.028, -107.872)
  line L5061 (142.886, -108.473) -> (142.967, -108.418)
  line L5062 (144.313, -109.524) -> (143.063, -109.524)
  line L5063 (144.578, -107.999) -> (144.451, -107.999)
  line L5064 (130.91, -107.85) -> (130.966, -107.85)
  line L5065 (145.303, -108.066) -> (145.281, -108.109)
  line L5066 (144.334, -107.768) -> (144.339, -107.764)
  line L5067 (144.331, -107.769) -> (144.334, -107.768)
  line L5068 (144.834, -107.493) -> (144.958, -107.474)
  line L5069 (130.993, -107.853) -> (130.996, -107.855)
  line L5070 (132.578, -108.399) -> (132.674, -108.418)
  line L5071 (144.313, -108.399) -> (144.408, -108.418)
  line L5072 (144.369, -107.757) -> (144.399, -107.749)
  line L5073 (144.408, -108.418) -> (144.49, -108.473)
  line L5074 (143.063, -108.399) -> (143.697, -108.399)
  line L5075 (130.766, -107.652) -> (130.854, -107.74)
  line L5076 (130.996, -107.855) -> (131.002, -107.856)
  line L5077 (131.055, -107.887) -> (131.567, -108.399)
  line L5078 (130.854, -107.74) -> (130.91, -107.85)
  line L5079 (144.399, -107.749) -> (144.578, -107.749)
  line L5080 (145.193, -108.197) -> (145.081, -108.254)
  line L5081 (142.967, -108.418) -> (143.063, -108.399)
  line L5082 (145.482, -108.418) -> (145.577, -108.399)
  line L5083 (144.723, -107.55) -> (144.834, -107.493)
  line L5084 (131.233, -108.418) -> (130.915, -108.1)
  line L5085 (132.755, -109.451) -> (132.674, -109.505)
  line L5086 (131.232, -109.505) -> (131.151, -109.451)
  line L5087 (131.078, -109.274) -> (131.078, -108.649)
  line L5088 (130.295, -108.299) -> (130.207, -108.211)
  line L5089 (132.674, -108.418) -> (132.755, -108.473)
  line L5090 (132.809, -109.37) -> (132.755, -109.451)
  line L5091 (132.755, -108.473) -> (132.809, -108.554)
  line L5092 (132.674, -109.505) -> (132.578, -109.524)
  line L5093 (130.854, -108.211) -> (130.766, -108.299)
  line L5094 (130.291, -109.451) -> (130.21, -109.505)
  line L5095 (130.194, -108.184) -> (129.979, -108.399)
  line L5096 (130.146, -107.881) -> (130.15, -107.852)
  line L5097 (132.809, -108.554) -> (132.828, -108.649)
  line L5098 (128.633, -108.554) -> (128.687, -108.473)
  line L5099 (131.151, -109.451) -> (131.097, -109.37)
  line L5100 (131.328, -109.524) -> (131.232, -109.505)
  line L5101 (132.828, -108.649) -> (132.828, -109.274)
  line L5102 (131.232, -108.418) -> (131.233, -108.418)
  line L5103 (132.578, -109.524) -> (131.328, -109.524)
  line L5104 (131.097, -109.37) -> (131.078, -109.274)
  line L5105 (131.078, -108.649) -> (131.097, -108.554)
  line L5106 (130.207, -108.211) -> (130.194, -108.184)
  line L5107 (131.151, -108.473) -> (131.232, -108.418)
  line L5108 (130.654, -108.356) -> (130.531, -108.375)
  line L5109 (130.295, -107.652) -> (130.407, -107.595)
  line L5110 (130.531, -108.375) -> (130.407, -108.356)
  line L5111 (130.407, -108.356) -> (130.295, -108.299)
  line L5112 (130.766, -108.299) -> (130.654, -108.356)
  line L5113 (131.097, -108.554) -> (131.151, -108.473)
  line L5114 (130.21, -108.418) -> (130.291, -108.473)
  line L5115 (128.864, -109.524) -> (128.769, -109.505)
  line L5116 (110.712, -108.02) -> (110.768, -108.13)
  line L5117 (129.625, -108.399) -> (130.137, -107.887)
  line L5118 (130.21, -109.505) -> (130.114, -109.524)
  line L5119 (130.114, -108.399) -> (130.21, -108.418)
  line L5120 (130.91, -108.1) -> (130.854, -108.211)
  line L5121 (132.828, -109.274) -> (132.809, -109.37)
  line L5122 (110.936, -108.13) -> (110.959, -108.133)
  line L5123 (110.959, -108.133) -> (110.963, -108.133)
  line L5124 (130.915, -108.1) -> (130.91, -108.1)
  line L5125 (130.345, -109.37) -> (130.291, -109.451)
  line L5126 (130.531, -107.575) -> (130.654, -107.595)
  line L5127 (112.435, -108.462) -> (112.489, -108.543)
  line L5128 (110.912, -108.408) -> (110.913, -108.408)
  line L5129 (130.291, -108.473) -> (130.345, -108.554)
  line L5130 (128.687, -109.451) -> (128.633, -109.37)
  line L5131 (110.712, -108.49) -> (110.624, -108.578)
  line L5132 (110.512, -108.635) -> (110.388, -108.655)
  line L5133 (110.624, -108.578) -> (110.512, -108.635)
  line L5134 (110.388, -108.655) -> (110.265, -108.635)
  line L5135 (110.768, -108.13) -> (110.936, -108.13)
  line L5136 (128.769, -108.418) -> (128.864, -108.399)
  line L5137 (130.345, -108.554) -> (130.364, -108.649)
  line L5138 (128.769, -109.505) -> (128.687, -109.451)
  line L5139 (128.687, -108.473) -> (128.769, -108.418)
  line L5140 (130.407, -107.595) -> (130.531, -107.575)
  line L5141 (130.207, -107.74) -> (130.295, -107.652)
  line L5142 (130.15, -107.852) -> (130.207, -107.74)
  line L5143 (130.114, -109.524) -> (128.864, -109.524)
  line L5144 (110.624, -107.931) -> (110.712, -108.02)
  line L5145 (112.508, -109.264) -> (112.489, -109.359)
  line L5146 (128.614, -109.274) -> (128.614, -108.649)
  line L5147 (112.435, -109.441) -> (112.354, -109.495)
  line L5148 (111.008, -109.514) -> (110.912, -109.495)
  line L5149 (110.768, -108.38) -> (110.712, -108.49)
  line L5150 (128.864, -108.399) -> (129.625, -108.399)
  line L5151 (128.633, -109.37) -> (128.614, -109.274)
  line L5152 (110.912, -109.495) -> (110.831, -109.441)
  line L5153 (110.963, -108.133) -> (110.966, -108.134)
  line L5154 (112.489, -109.359) -> (112.435, -109.441)
  line L5155 (112.258, -109.514) -> (111.008, -109.514)
  line L5156 (130.364, -109.274) -> (130.345, -109.37)
  line L5157 (110.998, -108.152) -> (111.025, -108.166)
  line L5158 (130.364, -108.649) -> (130.364, -109.274)
  line L5159 (110.777, -108.543) -> (110.831, -108.462)
  line L5160 (128.614, -108.649) -> (128.633, -108.554)
  line L5161 (110.512, -107.874) -> (110.624, -107.931)
  line L5162 (112.354, -109.495) -> (112.258, -109.514)
  line L5163 (110.972, -108.135) -> (110.998, -108.152)
  line L5164 (112.258, -108.389) -> (112.354, -108.408)
  line L5165 (110.966, -108.134) -> (110.972, -108.135)
  line L5166 (110.913, -108.408) -> (110.885, -108.38)
  line L5167 (111.025, -108.166) -> (111.247, -108.389)
  line L5168 (130.137, -107.887) -> (130.146, -107.881)
  line L5169 (110, -108.543) -> (110.019, -108.639)
  line L5170 (108.519, -109.514) -> (108.423, -109.495)
  line L5171 (112.508, -108.639) -> (112.508, -109.264)
  line L5172 (108.342, -109.441) -> (108.288, -109.359)
  line L5173 (110.019, -108.639) -> (110.019, -109.264)
  line L5174 (109.769, -109.514) -> (108.519, -109.514)
  line L5175 (110.265, -108.635) -> (110.153, -108.578)
  line L5176 (110, -109.359) -> (109.946, -109.441)
  line L5177 (110.265, -107.874) -> (110.388, -107.855)
  line L5178 (110.153, -108.578) -> (110.065, -108.49)
  line L5179 (110.885, -108.38) -> (110.768, -108.38)
  line L5180 (110.019, -109.264) -> (110, -109.359)
  line L5181 (109.864, -108.408) -> (109.946, -108.462)
  line L5182 (109.864, -109.495) -> (109.769, -109.514)
  line L5183 (110.758, -109.264) -> (110.758, -108.639)
  line L5184 (109.752, -108.166) -> (109.77, -108.153)
  line L5185 (109.864, -108.408) -> (109.864, -108.408)
  line L5186 (109.811, -108.138) -> (109.84, -108.13)
  line L5187 (108.342, -108.462) -> (108.423, -108.408)
  line L5188 (110.831, -109.441) -> (110.777, -109.359)
  line L5189 (108.423, -109.495) -> (108.342, -109.441)
  line L5190 (109.775, -108.149) -> (109.781, -108.145)
  line L5191 (109.53, -108.389) -> (109.752, -108.166)
  line L5192 (109.773, -108.15) -> (109.775, -108.149)
  line L5193 (110.758, -108.639) -> (110.777, -108.543)
  line L5194 (110.831, -108.462) -> (110.912, -108.408)
  line L5195 (112.489, -108.543) -> (112.508, -108.639)
  line L5196 (111.247, -108.389) -> (112.258, -108.389)
  line L5197 (110.777, -109.359) -> (110.758, -109.264)
  line L5198 (109.781, -108.145) -> (109.811, -108.138)
  line L5199 (112.354, -108.408) -> (112.435, -108.462)
  line L5200 (110.065, -108.49) -> (110.009, -108.38)
  line L5201 (108.519, -108.389) -> (109.53, -108.389)
  line L5202 (109.946, -108.462) -> (110, -108.543)
  line L5203 (108.288, -108.543) -> (108.342, -108.462)
  line L5204 (109.946, -109.441) -> (109.864, -109.495)
  line L5205 (109.77, -108.153) -> (109.773, -108.15)
  line L5206 (108.269, -108.639) -> (108.288, -108.543)
  line L5207 (108.269, -109.264) -> (108.269, -108.639)
  line L5208 (108.423, -108.408) -> (108.519, -108.389)
  line L5209 (109.892, -108.38) -> (109.864, -108.408)
  line L5210 (108.288, -109.359) -> (108.269, -109.264)
  line L5211 (110.009, -108.38) -> (109.892, -108.38)
  line L5212 (124.129, -108.12) -> (124.072, -108.231)
  line L5213 (123.361, -108.07) -> (123.26, -108.057)
  line L5214 (124.137, -109.359) -> (124.118, -109.264)
  line L5215 (124.57, -108.389) -> (124.238, -108.057)
  line L5216 (123.425, -108.231) -> (123.368, -108.12)
  line L5217 (124.266, -107.801) -> (124.301, -107.801)
  line L5218 (124.371, -107.836) -> (124.923, -108.389)
  line L5219 (109.84, -108.13) -> (110.009, -108.13)
  line L5220 (110.065, -108.02) -> (110.153, -107.931)
  line L5221 (124.309, -107.802) -> (124.337, -107.818)
  line L5222 (110.153, -107.931) -> (110.265, -107.874)
  line L5223 (125.795, -108.462) -> (125.849, -108.543)
  line L5224 (124.305, -107.803) -> (124.309, -107.802)
  line L5225 (125.849, -108.543) -> (125.868, -108.639)
  line L5226 (125.849, -109.359) -> (125.795, -109.441)
  line L5227 (125.714, -108.408) -> (125.795, -108.462)
  line L5228 (124.367, -107.834) -> (124.371, -107.836)
  line L5229 (110.388, -107.855) -> (110.512, -107.874)
  line L5230 (125.714, -109.495) -> (125.618, -109.514)
  line L5231 (124.365, -107.831) -> (124.367, -107.834)
  line L5232 (125.868, -108.639) -> (125.868, -109.264)
  line L5233 (125.795, -109.441) -> (125.714, -109.495)
  line L5234 (124.192, -109.441) -> (124.137, -109.359)
  line L5235 (124.273, -109.495) -> (124.192, -109.441)
  line L5236 (123.411, -108.543) -> (123.43, -108.639)
  line L5237 (124.072, -107.761) -> (124.104, -107.822)
  line L5238 (125.868, -109.264) -> (125.849, -109.359)
  line L5239 (123.872, -108.376) -> (123.749, -108.396)
  line L5240 (124.137, -108.07) -> (124.129, -108.12)
  line L5241 (124.301, -107.801) -> (124.305, -107.803)
  line L5242 (124.923, -108.389) -> (125.618, -108.389)
  line L5243 (124.337, -107.818) -> (124.365, -107.831)
  line L5244 (123.984, -107.672) -> (124.072, -107.761)
  line L5245 (123.26, -108.057) -> (122.928, -108.389)
  line L5246 (124.273, -108.408) -> (124.368, -108.389)
  line L5247 (110.009, -108.13) -> (110.065, -108.02)
  line L5248 (124.104, -107.822) -> (124.266, -107.801)
  line L5249 (123.872, -107.616) -> (123.984, -107.672)
  line L5250 (125.618, -109.514) -> (124.368, -109.514)
  line L5251 (124.072, -108.231) -> (123.984, -108.32)
  line L5252 (124.368, -109.514) -> (124.273, -109.495)
  line L5253 (125.618, -108.389) -> (125.714, -108.408)
  line L5254 (123.625, -108.376) -> (123.514, -108.32)
  line L5255 (123.228, -107.801) -> (123.232, -107.801)
  line L5256 (121.834, -108.408) -> (121.93, -108.389)
  line L5257 (121.93, -109.514) -> (121.834, -109.495)
  line L5258 (121.753, -108.462) -> (121.834, -108.408)
  line L5259 (122.928, -108.389) -> (123.18, -108.389)
  line L5260 (123.276, -109.495) -> (123.18, -109.514)
  line L5261 (123.749, -107.596) -> (123.872, -107.616)
  line L5262 (123.749, -108.396) -> (123.625, -108.376)
  line L5263 (124.118, -109.264) -> (124.118, -108.639)
  line L5264 (123.357, -109.441) -> (123.276, -109.495)
  line L5265 (123.156, -107.815) -> (123.16, -107.814)
  line L5266 (123.162, -107.811) -> (123.194, -107.807)
  line L5267 (121.834, -109.495) -> (121.753, -109.441)
  line L5268 (121.699, -108.543) -> (121.753, -108.462)
  line L5269 (123.357, -108.462) -> (123.411, -108.543)
  line L5270 (124.238, -108.057) -> (124.137, -108.07)
  line L5271 (123.514, -107.672) -> (123.625, -107.616)
  line L5272 (123.43, -109.264) -> (123.411, -109.359)
  line L5273 (123.18, -109.514) -> (121.93, -109.514)
  line L5274 (123.625, -107.616) -> (123.749, -107.596)
  line L5275 (123.514, -108.32) -> (123.425, -108.231)
  line L5276 (127.654, -107.061) -> (127.634, -107.185)
  line L5277 (123.18, -108.389) -> (123.276, -108.408)
  line L5278 (124.118, -108.639) -> (124.137, -108.543)
  line L5279 (121.68, -108.639) -> (121.699, -108.543)
  line L5280 (123.43, -108.639) -> (123.43, -109.264)
  line L5281 (121.93, -108.389) -> (122.574, -108.389)
  line L5282 (121.699, -109.359) -> (121.68, -109.264)
  line L5283 (123.232, -107.801) -> (123.394, -107.822)
  line L5284 (123.394, -107.822) -> (123.425, -107.761)
  line L5285 (127.578, -107.296) -> (127.489, -107.385)
  line L5286 (122.574, -108.389) -> (123.127, -107.836)
  line L5287 (123.276, -108.408) -> (123.357, -108.462)
  line L5288 (123.984, -108.32) -> (123.872, -108.376)
  line L5289 (127.638, -106.96) -> (127.654, -107.061)
  line L5290 (124.137, -108.543) -> (124.192, -108.462)
  line L5291 (124.192, -108.462) -> (124.273, -108.408)
  line L5292 (123.425, -107.761) -> (123.514, -107.672)
  line L5293 (121.68, -109.264) -> (121.68, -108.639)
  line L5294 (124.368, -108.389) -> (124.57, -108.389)
  line L5295 (123.411, -109.359) -> (123.357, -109.441)
  line L5296 (127.634, -107.185) -> (127.578, -107.296)
  line L5297 (123.368, -108.12) -> (123.361, -108.07)
  line L5298 (137.46, -111.947) -> (137.452, -111.949)
  line L5299 (137.47, -110.771) -> (137.472, -110.779)
  line L5300 (142.886, -111.398) -> (142.967, -111.343)
  line L5301 (143.063, -111.324) -> (144.313, -111.324)
  line L5302 (145.438, -112.777) -> (145.465, -112.83)
  line L5303 (144.501, -113.13) -> (144.479, -113.126)
  line L5304 (146.923, -112.43) -> (146.827, -112.449)
  line L5305 (142.813, -112.199) -> (142.813, -111.574)
  line L5306 (142.967, -112.43) -> (142.886, -112.376)
  line L5307 (145.208, -113.334) -> (145.085, -113.354)
  line L5308 (144.439, -113.108) -> (144.412, -113.093)
  line L5309 (144.465, -113.124) -> (144.439, -113.108)
  line L5310 (136.796, -112.602) -> (136.793, -112.603)
  line L5311 (144.471, -113.125) -> (144.465, -113.124)
  line L5312 (147.004, -112.376) -> (146.923, -112.43)
  line L5313 (137.397, -111.953) -> (137.394, -111.975)
  line L5314 (136.788, -112.606) -> (136.758, -112.613)
  line L5315 (137.394, -111.979) -> (137.393, -111.982)
  line L5316 (142.886, -112.376) -> (142.832, -112.295)
  line L5317 (137.375, -112.014) -> (137.36, -112.041)
  line L5318 (136.799, -112.598) -> (136.796, -112.602)
  line L5319 (136.176, -112.622) -> (136.176, -112.681)
  line L5320 (144.731, -113.13) -> (144.501, -113.13)
  line L5321 (136.817, -112.585) -> (136.799, -112.598)
  line L5322 (144.761, -113.189) -> (144.731, -113.13)
  line L5323 (143.063, -112.449) -> (142.967, -112.43)
  line L5324 (142.813, -111.574) -> (142.832, -111.479)
  line L5325 (143.769, -112.449) -> (143.063, -112.449)
  line L5326 (137.466, -111.943) -> (137.46, -111.947)
  line L5327 (137.466, -110.765) -> (137.47, -110.771)
  line L5328 (137.394, -111.975) -> (137.394, -111.979)
  line L5329 (146.827, -112.449) -> (145.766, -112.449)
  line L5330 (144.313, -111.324) -> (144.408, -111.343)
  line L5331 (145.485, -112.954) -> (145.465, -113.077)
  line L5332 (136.728, -112.622) -> (136.176, -112.622)
  line L5333 (136.176, -112.681) -> (136.176, -112.693)
  line L5334 (137.47, -111.936) -> (137.466, -111.943)
  line L5335 (137.397, -111.949) -> (137.397, -111.953)
  line L5336 (137.452, -111.949) -> (137.397, -111.949)
  line L5337 (142.967, -111.343) -> (143.063, -111.324)
  line L5338 (137.472, -111.929) -> (137.47, -111.936)
  line L5339 (142.832, -112.295) -> (142.813, -112.199)
  line L5340 (136.676, -112.372) -> (137.099, -111.949)
  line L5341 (135.75, -111.686) -> (135.886, -111.727)
  line L5342 (136.098, -111.912) -> (136.156, -112.041)
  line L5343 (137.074, -110.771) -> (137.078, -110.765)
  line L5344 (137.084, -111.947) -> (137.078, -111.943)
  line L5345 (135.676, -113.176) -> (135.676, -113.181)